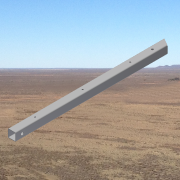
# Autodesk Inventor part: 2f2ax1
Saved by Autodesk Inventor 2014 SP1 (Build 180222100, 222)
## iProperties
Company: HERA Project
Created: 2013-06-27
Part Number: 2f2ax1
Material: Steel
Description: Feed backplane support interior piece
Document SubType Name: Modeling
Designer: David DeBoer
Mass: 156.218 g
Surface Area: 246.159 cm^2
Volume: 19.9004 cm^3
Density: 7.85 g/cm^3
Appearance: Steel
Title: Feed backplane support interior piece
Author: David DeBoer
Autodesk Inventor part; units mm, degrees
ref_plane "YZ Plane" through (0, 0, 0) normal (1, 0, 0) x (0, 1, 0)
ref_plane "XZ Plane" through (0, 0, 0) normal (0, 1, 0) x (-1, 0, 0)
ref_plane "XY Plane" through (0, 0, 0) normal (0, 0, 1) x (1, 0, 0)
sketch "Sketch1" plane through (0, 0, 0) normal (0, 0, 1) x (1, 0, 0)
  line L0 (3.7363, 0) -> (22.7863, 0)
  line L1 (25.9613, 3.175) -> (25.9613, 22.225)
  line L2 (22.7863, 25.4) -> (3.7363, 25.4)
  line L3 (0.5613, 22.225) -> (0.5613, 3.175)
  arc A0 (3.7363, 25.4) -> (0.5613, 22.225) centre (3.7363, 22.225) ccw
  arc A1 (0.5613, 3.175) -> (3.7363, 0) centre (3.7363, 3.175) ccw
  arc A2 (22.7863, 0) -> (25.9613, 3.175) centre (22.7863, 3.175) ccw
  arc A3 (25.9613, 22.225) -> (22.7863, 25.4) centre (22.7863, 22.225) ccw
  line L4 (3.7363, 23.749) -> (22.7863, 23.749)
  arc A4 (24.3103, 22.225) -> (22.7863, 23.749) centre (22.7863, 22.225) ccw
  line L5 (24.3103, 22.225) -> (24.3103, 3.175)
  arc A5 (22.7863, 1.651) -> (24.3103, 3.175) centre (22.7863, 3.175) ccw
  line L6 (22.7863, 1.651) -> (3.7363, 1.651)
  arc A6 (2.2123, 3.175) -> (3.7363, 1.651) centre (3.7363, 3.175) ccw
  line L7 (2.2123, 3.175) -> (2.2123, 22.225)
  arc A7 (3.7363, 23.749) -> (2.2123, 22.225) centre (3.7363, 22.225) ccw
  point P0 (0, 0)
  point P1 (0.5613, 0)
  point P2 (25.9613, 0)
  point P3 (0.5613, 25.4)
  dimension "d0" = 25.4
  dimension "d2" = 25.4
  dimension "d3" = 3.175
  dimension "d4" = 1.651
  constraints: 16 end point, 16 point on circle, 8 centre point, 8 tangent, 6 point on line, 4 parallel, 3 equal radius, 2 perpendicular, 1 horizontal, 7 other
  measures "d0" distance of point (0.561, 0) point (25.961, 0)
  measures "d2" distance of point (0.561, 25.4) point (0.561, 0)
  measures "d3" radius of A0
  measures "d4" distance between parallel lines of L4 L2
extrude "tube" add sketch "Sketch1" along normal blind 520.3
sketch "Sketch11" plane through (3.7363, 25.4, 0) normal (0, 1, 0) x (1, 0, 0)
  line L0 (19.05, 0) -> (0, 0) projected
  circle A0 centre (9.525, -20) radius 2.8743
  point P0 (-3.7363, 0)
  dimension "d83" = 20
  constraints: 1 centre point
  measures "d83" distance from line of A0.centre L0
hole "centerHole_cutOff" at (13.2613, 25.4, 20) direction (0, -1, 0) diameter 6.35 end through all
sketch "Sketch12" plane through (3.7363, 25.4, 0) normal (0, 1, 0) x (1, 0, 0)
  circle A0 centre (9.525, -20) radius 3.175 projected
  circle A1 centre (9.525, -77) radius 2.5235
  point P0 (-3.7363, 0)
  dimension "d91" = 57
  constraints: 1 centre point
  measures "d91" distance of A1.centre A0.centre
hole "collarHole" at (13.2613, 25.4, 77) direction (0, -1, 0) diameter 6.6 end through all clearance for "Hex Head Bolt" size "M6" standard "Ansi Metric M Profile"
sketch "Sketch8" plane through (3.7363, 25.4, 520.3) normal (0, 1, 0) x (1, 0, 0)
  line L0 (0, 520.3) -> (0, 0) projected
  circle A0 centre (9.525, 73.3) radius 1.5875
  circle A1 centre (9.525, 223.3) radius 1.5875
  circle A2 centre (9.525, 373.3) radius 1.5875
  circle A3 centre (9.525, 500.3) radius 3.175 projected
  point P0 (0, 518.1689)
  point P1 (-3.7363, 520.3)
  dimension "d43" = 3.175
  dimension "d47" = 150
  dimension "d99" = 127
  constraints: 3 centre point, 1 vertical, 4 other
  measures "d43" diameter of A0
  measures "d47" distance of A0.centre A1.centre
  measures "d99" distance of A2.centre A3.centre
hole "armAttach" at (13.2613, 25.4, 447) at (13.2613, 25.4, 297) at (13.2613, 25.4, 147) direction (0, -1, 0) diameter 4.5 end through all clearance for "Flat Head Machine Screw" size "M4" standard "Ansi Metric M Profile"
sketch "Sketch6" plane through (25.9613, 3.175, 520.3) normal (1, 0, 0) x (0, 0, -1)
  line L0 (0, 0) -> (0, 19.05) projected
  circle A0 centre (20, 9.525) radius 2.9685
  point P0 (520.3, -3.175)
  dimension "d27" = 20
  constraints: 1 centre point
  measures "d27" distance from line of A0.centre L0
hole "ropeAttach" at (25.9613, 12.7, 500.3) direction (-1, 0, 0) diameter 8 end through all
sketch "Sketch13" plane through (3.7363, 25.4, 0) normal (0, 1, 0) x (1, 0, 0)
  circle A0 centre (9.525, -20) radius 3.175 projected
  line L0 (9.525, -20) -> (9.525, -34.6812) construction
  line L1 (-12.9518, -21.6531) -> (31.0422, -47.0531)
  line L2 (0, -34.6812) -> (50.8, -34.6812) construction
  line L3 (-12.9518, 4.6365) -> (31.0422, 4.6365)
  line L4 (31.0422, -47.0531) -> (31.0422, 4.6365)
  line L5 (-12.9518, 4.6365) -> (-12.9518, -21.6531)
  point P0 (-3.7363, 0)
  dimension "d100" = 14.6812
  dimension "d101" = 50.8
  dimension "d102" = 30
  constraints: 12 end point, 1 equal length, 1 horizontal, 1 parallel, 1 perpendicular, 1 point on line
  measures "d100" distance of L0.start L0.end
  measures "d101" distance of L1.start L1.end
  measures "d102" angle of L1 L2
extrude "angledEnd" cut sketch "Sketch13" against normal blind 50.8
equation "\"d0\" = tube"
equation "\"d2\" = tube"
equation "\"tube\" = 25.4"
body "Solid1"
